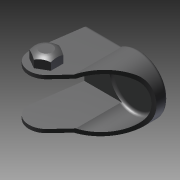
# Autodesk Inventor part: CHAMJ-E50-Rbody
Saved by Autodesk Inventor 2015 (Build 190159000, 159)
## iProperties
Category: PARTsolutions
Company: MISUMI
Created: 2015-12-24
Part Number: CHAMJ-E50-Rbody
Catalog Web Link: www.cadenas.de
Description: CHAMJ_E, CHAMK_E, CHAMS_Ebody-Caster
Vendor: MISUMI
Document SubType Name: Modeling
Designer: psAdmin
Manufacturer: MISUMI
Mass: 7.84838 g
Surface Area: 76.1016 cm^2
Volume: 7.84838 cm^3
Density: 1 g/cm^3
Material: 一般
Appearance: PSOLRGB-192-192-192
PSOL_IDENT_0: {$CADENAS_DATA\23d-libs\misumi\metric\42_casters_leveling_pads\chamj_e_body.prj},204 {VTYP=3D},{NB=C
PSOL_IDENT_1: HAMJ-E50-Rbody},{LINA=CHAMJ-E50-Rbody},{NN=CHAMJ_E, CHAMK_E, CHAMS_Ebody},{DATE=05.06.2015 05:25:12}
PSOL_IDENT_2: ,{GEOMDATE=03.09.2009 00:00:00},{VERSION=},{LINEID=30},{LINESUBID=-1},{WBVAR=TSMB,MATW}  {NB=CHAMJ-E
PSOL_IDENT_3: 50-Rbody},{LINA=CHAMJ-E50-Rbody},{KT=DUMMY},{PN=CHAMJ-E50-R},{TYPE=CHAMJ-E},{TSMB=1},{MATMB=Low Carb
PSOL_IDENT_4: on Steel},{STMB=Trivalnt Chromate},{D=50},{MATW=R},{COLORW=Black},{BSP=Available},{BWP=Not Available
PSOL_IDENT_5: },{H=65},{A=70},{C=42},{F1=56},{F2=28},{DD=6.5},{E=22},{RR=47},{B=20},{TT=2.0},{BR=20},{BU=21},{BN=2
PSOL_IDENT_6: 1},{AL=300},{ALR=300},{ALU=380},{ALN=400},{MASS=180}
NN: CHAMJ_E, CHAMK_E, CHAMS_Ebody
NT: Caster
NB: CHAMJ-E50-Rbody
NBSYN: $PN.body
LINA: CHAMJ-E50-Rbody
PN: CHAMJ-E50-R
TSMB: Swivel
MATMB: Low Carbon Steel
STMB: Trivalnt Chromate
D: 50
MATW: Synthetic Rubber
BSP: Available
BWP: Not Available
H: 65
A: 70
C: 42
F1: 56
F2: 28
DD: 6.5
TT: 2.0
BR: 20
BU: 21
BN: 21
ALR: 300
ALU: 380
ALN: 400
SUPPLIER: MISUMI
ARTICLENO: CHAMJ-E50-Rbody
BOMINFO: CHAMJ-E50-Rbody
CREATOR: CADENAS GmbH
Title: CHAMJ-E50-Rbody
Author: Cadenas PARTsolutions
Comments: Caster
Autodesk Inventor part; units mm, degrees
sketch "Sketch_1" plane through (0, 0, 0) normal (1, 0, 0) x (0, 1, 0)
  line L0 (-10, 0) -> (-50, 0)
  line L1 (-12, 0) -> (-12, 12)
  arc A0 (-12, 12) -> (-14, 14) centre (-14, 12) ccw
  line L2 (-14, 14) -> (-50, 14)
  line L3 (-50, 14) -> (-50, 16)
  line L4 (-50, 16) -> (-12, 16)
  arc A1 (-10, 14) -> (-12, 16) centre (-12, 14) ccw
  line L5 (-10, 14) -> (-10, 0)
  line L6 (-10, 0) -> (-12, 0)
  constraints: 14 end point, 4 point on circle, 2 centre point
revolve "Revolution1" add sketch "Sketch_1" angle 360 about axis through (0, -10, 0) along (0, -1, 0)
sketch "Sketch_3" plane through (0, 0, 0) normal (1, 0, 0) x (0, 1, 0)
  line L0 (-13, 14) -> (-78, 14)
  line L1 (-78, 14) -> (-78, 12)
  line L2 (-78, 12) -> (-13, 12)
  line L3 (-13, 12) -> (-13, -12)
  line L4 (-13, -12) -> (-78, -12)
  line L5 (-78, -12) -> (-78, -14)
  line L6 (-78, -14) -> (-13, -14)
  arc A0 (-13, -14) -> (-11, -12) centre (-13, -12) ccw
  line L7 (-11, -12) -> (-11, 12)
  arc A1 (-11, 12) -> (-13, 14) centre (-13, 12) ccw
  constraints: 16 end point, 4 point on circle, 2 centre point
extrude "Extrusion1" add sketch "Sketch_3" against normal blind 60
sketch "Sketch_17" plane through (0, 0, 0) normal (1, 0, 0) x (0, 1, 0)
  line L0 (-52, 0) -> (-12, 0)
  line L1 (-12, 0) -> (-12, -12)
  arc A0 (-14, -14) -> (-12, -12) centre (-14, -12) ccw
  line L2 (-14, -14) -> (-52, -14)
  line L3 (-52, -14) -> (-52, 0)
  line L4 (-52, 0) -> (-12, 0)
  constraints: 10 end point, 2 point on circle, 1 centre point
revolve "Revolution2" cut sketch "Sketch_17" angle 360 about axis through (0, -52, 0) along (0, -1, 0)
sketch "Sketch_15" plane through (0, 0, 0) normal (1, 0, 0) x (0, 1, 0)
  line L0 (-13, 12) -> (-80, 12)
  line L1 (-80, 12) -> (-80, -12)
  line L2 (-80, -12) -> (-13, -12)
  line L3 (-13, -12) -> (-13, 12)
  constraints: 8 end point
extrude "Extrusion2" cut sketch "Sketch_15" against normal blind 35
sketch "Sketch_6" plane through (0, 0, 0) normal (0, 0, 1) x (1, 0, 0)
  line L0 (-100, -200) -> (100, -200)
  line L1 (100, -200) -> (100, -16)
  line L2 (100, -16) -> (20.1753, -16)
  arc A0 (20.1753, -16) -> (9.2206, -20.7533) centre (20.1753, -31) ccw
  line L3 (9.2206, -20.7533) -> (-14.9502, -46.5942)
  arc A1 (-31.6532, -40) -> (-14.9502, -46.5942) centre (-22, -40) ccw
  line L4 (-31.6532, -40) -> (-26.1721, -1)
  line L5 (-26.1721, -1) -> (-100, -1)
  line L6 (-100, -1) -> (-100, -200)
  constraints: 14 end point, 4 point on circle, 2 centre point
extrude "Extrusion3" cut sketch "Sketch_6" along normal mid plane 140
sketch "Sketch_7" plane through (0, 0, -14) normal (0, 0, 1) x (1, 0, 0)
  circle A0 centre (-22, -40) radius 5
  constraints: 1 centre point
extrude "Extrusion4" add sketch "Sketch_7" against normal blind 2
sketch "Sketch_8" plane through (-22, 0, 0) normal (1, 0, 0) x (0, 0, -1)
  line L0 (-12, -40) -> (-20, -40)
  line L1 (-20, -40) -> (-20, -36.5)
  arc A0 (-18, -33) -> (-20, -36.5) centre (-10.4958, -39.6096) ccw
  line L2 (-18, -33) -> (-14, -33)
  line L3 (-14, -33) -> (-14, -35)
  line L4 (-14, -35) -> (-12, -35)
  line L5 (-12, -35) -> (-12, -40)
  line L6 (-12, -40) -> (-20, -40)
  constraints: 14 end point, 2 point on circle, 1 centre point
revolve "Revolution3" add sketch "Sketch_8" angle 360 about axis through (-22, -40, 12) along (0, 0, 1)
sketch "Sketch_10" plane through (0, 0, 14) normal (0, 0, 1) x (1, 0, 0)
  circle A0 centre (-22, -40) radius 9
  line L0 (-28, -36.5359) -> (-28, -43.4641)
  line L1 (-28, -43.4641) -> (-22, -46.9282)
  line L2 (-22, -46.9282) -> (-16, -43.4641)
  line L3 (-16, -43.4641) -> (-16, -36.5359)
  line L4 (-16, -36.5359) -> (-22, -33.0718)
  line L5 (-22, -33.0718) -> (-28, -36.5359)
  constraints: 12 end point, 1 centre point
extrude "Extrusion5" cut sketch "Sketch_10" along normal blind 10
ref_plane "body_to_bearing_XY" through (-22, -40, 0) normal (0, 0, 1) x (1, 0, 0)
ref_plane "body_to_bearing_YZ" through (-22, -40, 0) normal (1, 0, 0) x (0, 1, 0)
ref_plane "body_to_bearing_ZX" through (-22, -40, 0) normal (0, 1, 0) x (0, 0, 1)
ref_plane "body_to_dummy_XY" through (0, 0, 0) normal (0, 1, 0) x (1, 0, 0)
ref_plane "body_to_dummy_YZ" through (0, 0, 0) normal (1, 0, 0) x (0, 0, -1)
ref_plane "body_to_dummy_ZX" through (0, 0, 0) normal (0, 0, -1) x (0, 1, 0)
ref_plane "stopper_to_body_XY" through (-22, -40, 14) normal (0, 0, 1) x (1, 0, 0)
ref_plane "stopper_to_body_YZ" through (-22, -40, 14) normal (1, 0, 0) x (0, 1, 0)
ref_plane "stopper_to_body_ZX" through (-22, -40, 14) normal (0, 1, 0) x (0, 0, 1)
ref_plane "swivel_to_body_XY" through (0, -10, 0) normal (0, 1, 0) x (1, 0, 0)
ref_plane "swivel_to_body_YZ" through (0, -10, 0) normal (1, 0, 0) x (0, 0, -1)
ref_plane "swivel_to_body_ZX" through (0, -10, 0) normal (0, 0, -1) x (0, 1, 0)
body "Solid1"
